Autodesk Inventor part; units mm, degrees
(part 2 of 2)
  line L223 (5.6866, -31.9003) -> (4.2323, -29.1462)
  line L224 (4.2323, -29.1462) -> (3.6335, -32.1998)
  line L225 (3.6335, -32.1998) -> (2.9735, -32.296)
  line L226 (-1.0989, -28.5985) -> (2.0334, -28.5439)
  line L227 (2.0334, -28.5439) -> (2.046, -29.2642)
  spline S287 degree 2 poles (2.046, -29.2642) (1.714, -29.587) (1.1233, -30.1861) (0.8407, -30.5081) knots 0 0 0 1 2 2 2
  spline S288 degree 2 poles (0.8407, -30.5081) (0.2715, -31.1562) (-0.1391, -31.9291) (-0.132, -32.3366) knots 0 0 0 1 2 2 2
  spline S289 degree 2 poles (-0.132, -32.3366) (-0.1283, -32.5507) (0.009, -32.8694) (0.1302, -32.9703) knots 0 0 0 1 2 2 2
  spline S290 degree 2 poles (0.1302, -32.9703) (0.2514, -33.0711) (0.566, -33.1685) (0.7553, -33.1652) knots 0 0 0 1 2 2 2
  spline S291 degree 2 poles (0.7553, -33.1652) (0.9364, -33.1621) (1.3053, -33.065) (1.4728, -32.9921) knots 0 0 0 1 2 2 2
  spline S292 degree 2 poles (1.4728, -32.9921) (1.6159, -32.932) (1.8806, -32.7627) (1.9619, -32.7036) knots 0 0 0 1 2 2 2
  line L228 (1.9619, -32.7036) -> (1.9989, -32.703)
  line L229 (1.9989, -32.703) -> (2.0115, -33.4274)
  spline S293 degree 2 poles (2.0115, -33.4274) (1.8034, -33.534) (1.0537, -33.7488) (0.7162, -33.7547) knots 0 0 0 1 2 2 2
  spline S294 degree 2 poles (0.7162, -33.7547) (0.0041, -33.7671) (-0.8117, -33.0278) (-0.8229, -32.3857) knots 0 0 0 1 2 2 2
  spline S295 degree 2 poles (-0.8229, -32.3857) (-0.8281, -32.0853) (-0.6969, -31.5807) (-0.5772, -31.3645) knots 0 0 0 1 2 2 2
  spline S296 degree 2 poles (-0.5772, -31.3645) (-0.4576, -31.1401) (-0.1071, -30.6975) (0.0868, -30.4841) knots 0 0 0 1 2 2 2
  spline S297 degree 2 poles (0.0868, -30.4841) (0.4018, -30.1287) (1.1749, -29.3659) (1.4057, -29.1436) knots 0 0 0 1 2 2 2
  line L230 (1.4057, -29.1436) -> (-1.0886, -29.1871)
  line L231 (-1.0886, -29.1871) -> (-1.0989, -28.5985)
  spline S298 degree 2 poles (-5.2095, -30.7189) (-5.0516, -29.3613) (-4.1145, -28.1813) (-3.2926, -28.2769) knots 0 0 0 1 2 2 2
  spline S299 degree 2 poles (-3.2926, -28.2769) (-2.4584, -28.3739) (-1.8281, -29.761) (-1.9827, -31.09) knots 0 0 0 1 2 2 2
  spline S300 degree 2 poles (-1.9827, -31.09) (-2.1415, -32.4558) (-3.0776, -33.6275) (-3.9037, -33.5315) knots 0 0 0 1 2 2 2
  spline S301 degree 2 poles (-3.9037, -33.5315) (-4.7337, -33.4349) (-5.3626, -32.0356) (-5.2095, -30.7189) knots 0 0 0 1 2 2 2
  spline S302 degree 2 poles (-4.1638, -29.2822) (-4.2909, -29.5202) (-4.4621, -30.2794) (-4.5225, -30.7988) knots 0 0 0 1 2 2 2
  spline S303 degree 2 poles (-4.5225, -30.7988) (-4.5829, -31.3181) (-4.59, -32.0923) (-4.5178, -32.3618) knots 0 0 0 1 2 2 2
  spline S304 degree 2 poles (-4.5178, -32.3618) (-4.4455, -32.6313) (-4.1207, -32.9384) (-3.8385, -32.9712) knots 0 0 0 1 2 2 2
  spline S305 degree 2 poles (-3.8385, -32.9712) (-3.5564, -33.0041) (-3.1615, -32.7806) (-3.0243, -32.5272) knots 0 0 0 1 2 2 2
  spline S306 degree 2 poles (-3.0243, -32.5272) (-2.8921, -32.2814) (-2.7272, -31.5049) (-2.6696, -31.0101) knots 0 0 0 1 2 2 2
  spline S307 degree 2 poles (-2.6696, -31.0101) (-2.6078, -30.4785) (-2.5905, -29.7594) (-2.6645, -29.469) knots 0 0 0 1 2 2 2
  spline S308 degree 2 poles (-2.6645, -29.469) (-2.7322, -29.1958) (-3.0633, -28.8714) (-3.3577, -28.8371) knots 0 0 0 1 2 2 2
  spline S309 degree 2 poles (-3.3577, -28.8371) (-3.6358, -28.8048) (-4.0306, -29.0283) (-4.1638, -29.2822) knots 0 0 0 1 2 2 2
  line L232 (-8.5894, -27.3003) -> (-5.5532, -28.0722)
  line L233 (-5.5532, -28.0722) -> (-5.7307, -28.7704)
  spline S310 degree 2 poles (-5.7307, -28.7704) (-6.136, -28.9945) (-6.8636, -29.4169) (-7.221, -29.6531) knots 0 0 0 1 2 2 2
  spline S311 degree 2 poles (-7.221, -29.6531) (-7.9407, -30.1285) (-8.5404, -30.7661) (-8.6408, -31.1611) knots 0 0 0 1 2 2 2
  spline S312 degree 2 poles (-8.6408, -31.1611) (-8.6936, -31.3685) (-8.645, -31.7122) (-8.5547, -31.8414) knots 0 0 0 1 2 2 2
  spline S313 degree 2 poles (-8.5547, -31.8414) (-8.4643, -31.9705) (-8.1865, -32.1474) (-8.0029, -32.194) knots 0 0 0 1 2 2 2
  spline S314 degree 2 poles (-8.0029, -32.194) (-7.8274, -32.2387) (-7.446, -32.2422) (-7.2652, -32.216) knots 0 0 0 1 2 2 2
  spline S315 degree 2 poles (-7.2652, -32.216) (-7.1113, -32.1956) (-6.8114, -32.1019) (-6.7174, -32.0664) knots 0 0 0 1 2 2 2
  line L234 (-6.7174, -32.0664) -> (-6.6815, -32.0755)
  line L235 (-6.6815, -32.0755) -> (-6.86, -32.7777)
  spline S316 degree 2 poles (-6.86, -32.7777) (-7.0889, -32.8257) (-7.8687, -32.8356) (-8.1959, -32.7524) knots 0 0 0 1 2 2 2
  spline S317 degree 2 poles (-8.1959, -32.7524) (-8.8861, -32.5769) (-9.4785, -31.649) (-9.3202, -31.0266) knots 0 0 0 1 2 2 2
  spline S318 degree 2 poles (-9.3202, -31.0266) (-9.2462, -30.7353) (-8.9867, -30.283) (-8.8143, -30.106) knots 0 0 0 1 2 2 2
  spline S319 degree 2 poles (-8.8143, -30.106) (-8.6398, -29.921) (-8.1852, -29.5863) (-7.942, -29.4316) knots 0 0 0 1 2 2 2
  spline S320 degree 2 poles (-7.942, -29.4316) (-7.5445, -29.1715) (-6.5979, -28.6392) (-6.3167, -28.4855) knots 0 0 0 1 2 2 2
  line L236 (-6.3167, -28.4855) -> (-8.7345, -27.8708)
  line L237 (-8.7345, -27.8708) -> (-8.5894, -27.3003)
  spline S321 degree 2 poles (-13.1132, -28.2636) (-12.6035, -26.9955) (-11.3888, -26.1039) (-10.621, -26.4125) knots 0 0 0 1 2 2 2
  spline S322 degree 2 poles (-10.621, -26.4125) (-9.8418, -26.7257) (-9.599, -28.2298) (-10.098, -29.4712) knots 0 0 0 1 2 2 2
  spline S323 degree 2 poles (-10.098, -29.4712) (-10.6108, -30.7469) (-11.8224, -31.6309) (-12.5939, -31.3208) knots 0 0 0 1 2 2 2
  spline S324 degree 2 poles (-12.5939, -31.3208) (-13.3693, -31.0091) (-13.6076, -29.4935) (-13.1132, -28.2636) knots 0 0 0 1 2 2 2
  spline S325 degree 2 poles (-11.7262, -27.1529) (-11.9115, -27.349) (-12.2765, -28.0364) (-12.4715, -28.5215) knots 0 0 0 1 2 2 2
  spline S326 degree 2 poles (-12.4715, -28.5215) (-12.6665, -29.0066) (-12.8772, -29.7516) (-12.8784, -30.0306) knots 0 0 0 1 2 2 2
  spline S327 degree 2 poles (-12.8784, -30.0306) (-12.8797, -30.3097) (-12.6472, -30.6915) (-12.3836, -30.7975) knots 0 0 0 1 2 2 2
  spline S328 degree 2 poles (-12.3836, -30.7975) (-12.1201, -30.9034) (-11.6803, -30.7918) (-11.4812, -30.5834) knots 0 0 0 1 2 2 2
  spline S329 degree 2 poles (-11.4812, -30.5834) (-11.289, -30.3811) (-10.9254, -29.6754) (-10.7397, -29.2132) knots 0 0 0 1 2 2 2
  spline S330 degree 2 poles (-10.7397, -29.2132) (-10.5401, -28.7167) (-10.334, -28.0275) (-10.3289, -27.7278) knots 0 0 0 1 2 2 2
  spline S331 degree 2 poles (-10.3289, -27.7278) (-10.3224, -27.4465) (-10.5564, -27.0463) (-10.8314, -26.9358) knots 0 0 0 1 2 2 2
  spline S332 degree 2 poles (-10.8314, -26.9358) (-11.0911, -26.8314) (-11.5309, -26.943) (-11.7262, -27.1529) knots 0 0 0 1 2 2 2
  line L238 (-24.6036, 2.7427) -> (-24.6056, 2.7098)
  spline S333 degree 2 poles (-24.6056, 2.7098) (-24.6436, 2.6255) (-24.7201, 2.3083) (-24.7276, 2.1809) knots 0 0 0 1 2 2 2
  spline S334 degree 2 poles (-24.7276, 2.1809) (-24.7514, 1.7782) (-24.4102, 1.4116) (-23.9335, 1.3834) knots 0 0 0 1 2 2 2
  line L239 (-23.9335, 1.3834) -> (-23.8061, 1.3759)
  line L240 (-23.8061, 1.3759) -> (-23.7434, 2.4361)
  line L241 (-23.7434, 2.4361) -> (-23.2133, 2.4047)
  line L242 (-23.2133, 2.4047) -> (-23.2748, 1.365)
  line L243 (-23.2748, 1.365) -> (-19.9995, 1.1712)
  line L244 (-19.9995, 1.1712) -> (-20.0375, 0.5301)
  line L245 (-20.0375, 0.5301) -> (-23.3127, 0.724)
  line L246 (-23.3127, 0.724) -> (-23.3383, 0.2925)
  line L247 (-23.3383, 0.2925) -> (-23.8684, 0.3238)
  line L248 (-23.8684, 0.3238) -> (-23.8429, 0.7553)
  line L249 (-23.8429, 0.7553) -> (-23.9703, 0.7629)
  spline S335 degree 2 poles (-23.9703, 0.7629) (-24.6524, 0.8032) (-25.3283, 1.5072) (-25.2918, 2.1236) knots 0 0 0 1 2 2 2
  spline S336 degree 2 poles (-25.2918, 2.1236) (-25.2814, 2.3003) (-25.2242, 2.6392) (-25.1913, 2.7775) knots 0 0 0 1 2 2 2
  line L250 (-25.1913, 2.7775) -> (-24.6036, 2.7427)
  line L251 (-19.7335, 3.4706) -> (-19.8346, 2.8364)
  line L252 (-19.8346, 2.8364) -> (-23.5991, 3.4365)
  line L253 (-23.5991, 3.4365) -> (-23.498, 4.0707)
  line L254 (-23.498, 4.0707) -> (-19.7335, 3.4706)
  line L255 (-24.117, 4.2152) -> (-24.2317, 3.4956)
  line L256 (-24.2317, 3.4956) -> (-24.8902, 3.6006)
  line L257 (-24.8902, 3.6006) -> (-24.7755, 4.3201)
  line L258 (-24.7755, 4.3201) -> (-24.117, 4.2152)
  line L259 (-19.3946, 5.0304) -> (-19.5458, 4.4063)
  line L260 (-19.5458, 4.4063) -> (-24.703, 5.6561)
  line L261 (-24.703, 5.6561) -> (-24.5517, 6.2802)
  line L262 (-24.5517, 6.2802) -> (-19.3946, 5.0304)
  spline S337 degree 2 poles (-18.5023, 7.4594) (-18.832, 6.607) (-20.1504, 6.04) (-21.0334, 6.3816) knots 0 0 0 1 2 2 2
  spline S338 degree 2 poles (-21.0334, 6.3816) (-21.9012, 6.7172) (-22.5781, 8.0252) (-22.2945, 8.7585) knots 0 0 0 1 2 2 2
  spline S339 degree 2 poles (-22.2945, 8.7585) (-22.1668, 9.0887) (-21.7773, 9.5251) (-21.501, 9.6345) knots 0 0 0 1 2 2 2
  spline S340 degree 2 poles (-21.501, 9.6345) (-21.2232, 9.7478) (-20.5571, 9.7241) (-20.1309, 9.5592) knots 0 0 0 1 2 2 2
  line L263 (-20.1309, 9.5592) -> (-19.8046, 9.433)
  line L264 (-19.8046, 9.433) -> (-20.7566, 6.9719)
  spline S341 degree 2 poles (-20.7566, 6.9719) (-20.1384, 6.7328) (-19.2413, 7.1008) (-19.0274, 7.6537) knots 0 0 0 1 2 2 2
  spline S342 degree 2 poles (-19.0274, 7.6537) (-18.9516, 7.8495) (-18.8929, 8.2637) (-18.9026, 8.4441) knots 0 0 0 1 2 2 2
  spline S343 degree 2 poles (-18.9026, 8.4441) (-18.917, 8.635) (-18.9653, 8.9097) (-18.9985, 9.0064) knots 0 0 0 1 2 2 2
  line L265 (-18.9985, 9.0064) -> (-18.9851, 9.0409)
  line L266 (-18.9851, 9.0409) -> (-18.3324, 8.7885)
  spline S344 degree 2 poles (-18.3324, 8.7885) (-18.3303, 8.6685) (-18.3292, 8.3061) (-18.3422, 8.1699) knots 0 0 0 1 2 2 2
  spline S345 degree 2 poles (-18.3422, 8.1699) (-18.3591, 7.9778) (-18.4191, 7.6744) (-18.5023, 7.4594) knots 0 0 0 1 2 2 2
  spline S346 degree 2 poles (-20.4872, 9.0261) (-20.7321, 9.112) (-21.1239, 9.1488) (-21.2801, 9.0988) knots 0 0 0 1 2 2 2
  spline S347 degree 2 poles (-21.2801, 9.0988) (-21.4545, 9.0472) (-21.7228, 8.7758) (-21.8164, 8.5339) knots 0 0 0 1 2 2 2
  spline S348 degree 2 poles (-21.8164, 8.5339) (-21.9085, 8.2958) (-21.8956, 7.9068) (-21.8109, 7.7152) knots 0 0 0 1 2 2 2
  spline S349 degree 2 poles (-21.8109, 7.7152) (-21.7208, 7.5258) (-21.4325, 7.2554) (-21.2134, 7.1486) knots 0 0 0 1 2 2 2
  line L267 (-21.2134, 7.1486) -> (-20.4872, 9.0261)
  line L268 (-17.161, 10.345) -> (-17.5675, 9.6386)
  line L269 (-17.5675, 9.6386) -> (-18.4096, 10.1231)
  line L270 (-18.4096, 10.1231) -> (-18.003, 10.8296)
  line L271 (-18.003, 10.8296) -> (-17.161, 10.345)
  line L272 (-19.623, 11.7618) -> (-20.0295, 11.0553)
  line L273 (-20.0295, 11.0553) -> (-20.8716, 11.5398)
  line L274 (-20.8716, 11.5398) -> (-20.465, 12.2463)
  line L275 (-20.465, 12.2463) -> (-19.623, 11.7618)
  spline S350 degree 2 poles (-14.6344, 12.8419) (-14.5674, 12.8679) (-14.3254, 12.9806) (-14.1854, 13.0675) knots 0 0 0 1 2 2 2
  spline S351 degree 2 poles (-14.1854, 13.0675) (-14.0279, 13.1602) (-13.777, 13.334) (-13.6514, 13.4588) knots 0 0 0 1 2 2 2
  spline S352 degree 2 poles (-13.6514, 13.4588) (-13.4412, 13.6677) (-13.2594, 14.0688) (-13.2763, 14.2494) knots 0 0 0 1 2 2 2
  spline S353 degree 2 poles (-13.2763, 14.2494) (-13.2961, 14.427) (-13.493, 14.7478) (-13.6584, 14.9143) knots 0 0 0 1 2 2 2
  line L276 (-13.6584, 14.9143) -> (-13.8934, 15.1508)
  spline S354 degree 2 poles (-13.8934, 15.1508) (-13.9178, 14.8074) (-14.1203, 14.3045) (-14.386, 14.0404) knots 0 0 0 1 2 2 2
  spline S355 degree 2 poles (-14.386, 14.0404) (-14.8474, 13.582) (-16.0754, 13.7256) (-16.7167, 14.371) knots 0 0 0 1 2 2 2
  spline S356 degree 2 poles (-16.7167, 14.371) (-17.0503, 14.7068) (-17.377, 15.4152) (-17.4021, 15.7559) knots 0 0 0 1 2 2 2
  spline S357 degree 2 poles (-17.4021, 15.7559) (-17.4215, 16.0791) (-17.1925, 16.6838) (-16.9705, 16.9043) knots 0 0 0 1 2 2 2
  spline S358 degree 2 poles (-16.9705, 16.9043) (-16.7603, 17.1132) (-16.355, 17.3186) (-16.1103, 17.3819) knots 0 0 0 1 2 2 2
  line L277 (-16.1103, 17.3819) -> (-16.1971, 17.5219)
  line L278 (-16.1971, 17.5219) -> (-15.7679, 17.9484)
  line L279 (-15.7679, 17.9484) -> (-13.3886, 15.5538)
  spline S359 degree 2 poles (-13.3886, 15.5538) (-12.7038, 14.8646) (-12.6641, 13.6274) (-13.2802, 13.0151) knots 0 0 0 1 2 2 2
  spline S360 degree 2 poles (-13.2802, 13.0151) (-13.4788, 12.8178) (-13.9573, 12.47) (-14.1877, 12.3456) knots 0 0 0 1 2 2 2
  line L280 (-14.1877, 12.3456) -> (-14.6578, 12.8187)
  line L281 (-14.6578, 12.8187) -> (-14.6344, 12.8419)
  line L282 (-14.2648, 15.5246) -> (-15.7418, 17.011)
  spline S361 degree 2 poles (-15.7418, 17.011) (-15.9924, 16.9245) (-16.3482, 16.7102) (-16.4913, 16.568) knots 0 0 0 1 2 2 2
  spline S362 degree 2 poles (-16.4913, 16.568) (-16.8359, 16.2256) (-16.7282, 15.3229) (-16.2552, 14.8469) knots 0 0 0 1 2 2 2
  spline S363 degree 2 poles (-16.2552, 14.8469) (-15.8084, 14.3972) (-15.0404, 14.2259) (-14.7017, 14.5625) knots 0 0 0 1 2 2 2
  spline S364 degree 2 poles (-14.7017, 14.5625) (-14.5235, 14.7395) (-14.289, 15.2511) (-14.2648, 15.5246) knots 0 0 0 1 2 2 2
  spline S365 degree 2 poles (-10.9409, 16.6815) (-11.6979, 16.1695) (-13.1042, 16.4559) (-13.6346, 17.2403) knots 0 0 0 1 2 2 2
  spline S366 degree 2 poles (-13.6346, 17.2403) (-14.1558, 18.011) (-13.9657, 19.4714) (-13.3144, 19.9119) knots 0 0 0 1 2 2 2
  spline S367 degree 2 poles (-13.3144, 19.9119) (-13.0211, 20.1102) (-12.4522, 20.2464) (-12.1629, 20.1787) knots 0 0 0 1 2 2 2
  spline S368 degree 2 poles (-12.1629, 20.1787) (-11.8702, 20.1133) (-11.3366, 19.7138) (-11.0806, 19.3352) knots 0 0 0 1 2 2 2
  line L283 (-11.0806, 19.3352) -> (-10.8846, 19.0454)
  line L284 (-10.8846, 19.0454) -> (-13.0705, 17.5671)
  spline S369 degree 2 poles (-13.0705, 17.5671) (-12.6992, 17.0181) (-11.7524, 16.8086) (-11.2613, 17.1407) knots 0 0 0 1 2 2 2
  spline S370 degree 2 poles (-11.2613, 17.1407) (-11.0874, 17.2583) (-10.8029, 17.565) (-10.708, 17.7187) knots 0 0 0 1 2 2 2
  spline S371 degree 2 poles (-10.708, 17.7187) (-10.6109, 17.8837) (-10.4938, 18.1368) (-10.4659, 18.2352) knots 0 0 0 1 2 2 2
  line L285 (-10.4659, 18.2352) -> (-10.4352, 18.256)
  line L286 (-10.4352, 18.256) -> (-10.0432, 17.6762)
  spline S372 degree 2 poles (-10.0432, 17.6762) (-10.1099, 17.5765) (-10.3157, 17.2782) (-10.4041, 17.1738) knots 0 0 0 1 2 2 2
  spline S373 degree 2 poles (-10.4041, 17.1738) (-10.5275, 17.0256) (-10.7499, 16.8107) (-10.9409, 16.6815) knots 0 0 0 1 2 2 2
  spline S374 degree 2 poles (-11.6774, 19.1007) (-11.8295, 19.3109) (-12.1303, 19.5646) (-12.287, 19.6127) knots 0 0 0 1 2 2 2
  spline S375 degree 2 poles (-12.287, 19.6127) (-12.4598, 19.6698) (-12.835, 19.5999) (-13.0499, 19.4547) knots 0 0 0 1 2 2 2
  spline S376 degree 2 poles (-13.0499, 19.4547) (-13.2613, 19.3117) (-13.4726, 18.9849) (-13.5124, 18.7791) knots 0 0 0 1 2 2 2
  spline S377 degree 2 poles (-13.5124, 18.7791) (-13.5464, 18.5722) (-13.4639, 18.1857) (-13.3449, 17.9729) knots 0 0 0 1 2 2 2
  line L287 (-13.3449, 17.9729) -> (-11.6774, 19.1007)
  spline S378 degree 2 poles (-7.4887, 19.0308) (-7.5373, 18.9466) (-7.6964, 18.6525) (-7.7848, 18.5465) knots 0 0 0 1 2 2 2
  spline S379 degree 2 poles (-7.7848, 18.5465) (-7.9032, 18.396) (-8.1558, 18.1823) (-8.4199, 18.0669) knots 0 0 0 1 2 2 2
  spline S380 degree 2 poles (-8.4199, 18.0669) (-8.6349, 17.973) (-9.0943, 17.9655) (-9.3057, 18.0484) knots 0 0 0 1 2 2 2
  spline S381 degree 2 poles (-9.3057, 18.0484) (-9.5079, 18.1307) (-9.8623, 18.4791) (-9.9644, 18.713) knots 0 0 0 1 2 2 2
  spline S382 degree 2 poles (-9.9644, 18.713) (-10.1226, 19.0752) (-10.0412, 19.7217) (-9.7735, 20.0138) knots 0 0 0 1 2 2 2
  spline S383 degree 2 poles (-9.7735, 20.0138) (-9.5385, 20.2782) (-8.7833, 20.7294) (-8.3308, 20.9585) knots 0 0 0 1 2 2 2
  line L288 (-8.3308, 20.9585) -> (-8.3802, 21.0717)
  spline S384 degree 2 poles (-8.3802, 21.0717) (-8.4692, 21.2754) (-8.7041, 21.4738) (-8.8486, 21.496) knots 0 0 0 1 2 2 2
  spline S385 degree 2 poles (-8.8486, 21.496) (-8.9931, 21.5182) (-9.3373, 21.4218) (-9.5108, 21.346) knots 0 0 0 1 2 2 2
  spline S386 degree 2 poles (-9.5108, 21.346) (-9.7145, 21.257) (-10.2126, 20.8957) (-10.4369, 20.6584) knots 0 0 0 1 2 2 2
  line L289 (-10.4369, 20.6584) -> (-10.4708, 20.6436)
  line L290 (-10.4708, 20.6436) -> (-10.7329, 21.2434)
  spline S387 degree 2 poles (-10.7329, 21.2434) (-10.5904, 21.3596) (-10.0325, 21.738) (-9.7345, 21.8682) knots 0 0 0 1 2 2 2
  spline S388 degree 2 poles (-9.7345, 21.8682) (-9.3723, 22.0264) (-8.8287, 22.1291) (-8.5682, 22.0677) knots 0 0 0 1 2 2 2
  spline S389 degree 2 poles (-8.5682, 22.0677) (-8.3132, 22.0084) (-7.9252, 21.6343) (-7.7818, 21.3061) knots 0 0 0 1 2 2 2
  line L291 (-7.7818, 21.3061) -> (-6.7387, 18.9181)
  line L292 (-6.7387, 18.9181) -> (-7.3272, 18.6611)
  line L293 (-7.3272, 18.6611) -> (-7.4887, 19.0308)
  line L294 (-7.7029, 19.5212) -> (-8.1264, 20.4907)
  spline S390 degree 2 poles (-8.1264, 20.4907) (-8.3295, 20.3796) (-8.939, 20.0369) (-9.1126, 19.8892) knots 0 0 0 1 2 2 2
  spline S391 degree 2 poles (-9.1126, 19.8892) (-9.3152, 19.7154) (-9.4905, 19.2839) (-9.3752, 19.0198) knots 0 0 0 1 2 2 2
  spline S392 degree 2 poles (-9.3752, 19.0198) (-9.2434, 18.718) (-8.7704, 18.5607) (-8.4459, 18.7025) knots 0 0 0 1 2 2 2
  spline S393 degree 2 poles (-8.4459, 18.7025) (-8.1705, 18.8228) (-7.8217, 19.2582) (-7.7029, 19.5212) knots 0 0 0 1 2 2 2
  line L295 (-4.717, 22.706) -> (-4.7489, 22.6976)
  spline S394 degree 2 poles (-4.7489, 22.6976) (-4.8258, 22.6986) (-4.9831, 22.6657) (-5.0906, 22.6373) knots 0 0 0 1 2 2 2
  spline S395 degree 2 poles (-5.0906, 22.6373) (-5.3414, 22.5712) (-5.7773, 22.2222) (-5.9435, 21.9485) knots 0 0 0 1 2 2 2
  line L296 (-5.9435, 21.9485) -> (-5.2541, 19.3331)
  line L297 (-5.2541, 19.3331) -> (-5.8751, 19.1694)
  line L298 (-5.8751, 19.1694) -> (-6.8468, 22.8556)
  line L299 (-6.8468, 22.8556) -> (-6.2258, 23.0193)
  line L300 (-6.2258, 23.0193) -> (-6.081, 22.4699)
  spline S396 degree 2 poles (-6.081, 22.4699) (-5.8224, 22.8617) (-5.3819, 23.2417) (-5.1431, 23.3047) knots 0 0 0 1 2 2 2
  spline S397 degree 2 poles (-5.1431, 23.3047) (-5.0475, 23.3299) (-4.9499, 23.3471) (-4.887, 23.3509) knots 0 0 0 1 2 2 2
  line L301 (-4.887, 23.3509) -> (-4.717, 22.706)
  line L302 (-0.4579, 20.1023) -> (-3.384, 19.7837)
  line L303 (-3.384, 19.7837) -> (-3.9339, 24.8339)
  line L304 (-3.9339, 24.8339) -> (-3.2628, 24.9069)
  line L305 (-3.2628, 24.9069) -> (-2.7779, 20.4543)
  line L306 (-2.7779, 20.4543) -> (-0.523, 20.6998)
  line L307 (-0.523, 20.6998) -> (-0.4579, 20.1023)
  spline S398 degree 2 poles (3.2846, 21.7592) (3.2149, 20.7985) (2.2151, 19.8184) (1.4432, 19.8744) knots 0 0 0 1 2 2 2
  spline S399 degree 2 poles (1.4432, 19.8744) (0.6508, 19.9319) (-0.1783, 21.0775) (-0.111, 22.0055) knots 0 0 0 1 2 2 2
  spline S400 degree 2 poles (-0.111, 22.0055) (-0.0419, 22.958) (0.9707, 23.9454) (1.7344, 23.89) knots 0 0 0 1 2 2 2
  spline S401 degree 2 poles (1.7344, 23.89) (2.5063, 23.834) (3.3539, 22.7159) (3.2846, 21.7592) knots 0 0 0 1 2 2 2
  spline S402 degree 2 poles (2.6235, 21.8072) (2.6771, 22.5462) (2.1913, 23.3038) (1.6945, 23.3398) knots 0 0 0 1 2 2 2
  spline S403 degree 2 poles (1.6945, 23.3398) (1.1977, 23.3758) (0.6036, 22.6966) (0.55, 21.9575) knots 0 0 0 1 2 2 2
  spline S404 degree 2 poles (0.55, 21.9575) (0.4979, 21.239) (0.9863, 20.4606) (1.4831, 20.4246) knots 0 0 0 1 2 2 2
  spline S405 degree 2 poles (1.4831, 20.4246) (1.9758, 20.3889) (2.5705, 21.0763) (2.6235, 21.8072) knots 0 0 0 1 2 2 2
  spline S406 degree 2 poles (5.2345, 19.2518) (4.8513, 19.3484) (4.276, 19.744) (4.1088, 20.0409) knots 0 0 0 1 2 2 2
  spline S407 degree 2 poles (4.1088, 20.0409) (3.9407, 20.3337) (3.8724, 21.1237) (3.9952, 21.6107) knots 0 0 0 1 2 2 2
  spline S408 degree 2 poles (3.9952, 21.6107) (4.118, 22.0976) (4.5566, 22.7427) (4.8366, 22.9269) knots 0 0 0 1 2 2 2
  spline S409 degree 2 poles (4.8366, 22.9269) (5.1175, 23.115) (5.8336, 23.2104) (6.2088, 23.1158) knots 0 0 0 1 2 2 2
  spline S410 degree 2 poles (6.2088, 23.1158) (6.5122, 23.0393) (7.0357, 22.7247) (7.2271, 22.5576) knots 0 0 0 1 2 2 2
  line L308 (7.2271, 22.5576) -> (7.051, 21.8591)
  line L309 (7.051, 21.8591) -> (7.015, 21.8681)
  spline S411 degree 2 poles (7.015, 21.8681) (6.9613, 21.9411) (6.7899, 22.1371) (6.6614, 22.2502) knots 0 0 0 1 2 2 2
  spline S412 degree 2 poles (6.6614, 22.2502) (6.5457, 22.3473) (6.2196, 22.5357) (6.06, 22.576) knots 0 0 0 1 2 2 2
  spline S413 degree 2 poles (6.06, 22.576) (5.577, 22.6977) (4.806, 22.1152) (4.6379, 21.4486) knots 0 0 0 1 2 2 2
  spline S414 degree 2 poles (4.6379, 21.4486) (4.4738, 20.7979) (4.8564, 19.9245) (5.3594, 19.7977) knots 0 0 0 1 2 2 2
  spline S415 degree 2 poles (5.3594, 19.7977) (5.6628, 19.7212) (6.277, 19.8338) (6.5379, 19.976) knots 0 0 0 1 2 2 2
  line L310 (6.5379, 19.976) -> (6.5739, 19.967)
  line L311 (6.5739, 19.967) -> (6.3977, 19.2684)
  spline S416 degree 2 poles (6.3977, 19.2684) (6.2948, 19.2477) (5.9842, 19.1944) (5.8654, 19.1946) knots 0 0 0 1 2 2 2
  spline S417 degree 2 poles (5.8654, 19.1946) (5.6936, 19.187) (5.4301, 19.2025) (5.2345, 19.2518) knots 0 0 0 1 2 2 2
  line L312 (9.7814, 17.5848) -> (9.0087, 17.9242)
  line L313 (9.0087, 17.9242) -> (8.4522, 20.1785)
  line L314 (8.4522, 20.1785) -> (8.1192, 20.055)
  line L315 (8.1192, 20.055) -> (7.4784, 18.5964)
  line L316 (7.4784, 18.5964) -> (6.8905, 18.8546)
  line L317 (6.8905, 18.8546) -> (9.0245, 23.713)
  line L318 (9.0245, 23.713) -> (9.6125, 23.4547)
  line L319 (9.6125, 23.4547) -> (8.3642, 20.6128)
  line L320 (8.3642, 20.6128) -> (10.391, 21.4806)
  line L321 (10.391, 21.4806) -> (11.1222, 21.1594)
  line L322 (11.1222, 21.1594) -> (9.0492, 20.3299)
  line L323 (9.0492, 20.3299) -> (9.7814, 17.5848)
  line L324 (10.8701, 16.8332) -> (10.1766, 17.2615)
  line L325 (10.1766, 17.2615) -> (10.6871, 18.0881)
  line L326 (10.6871, 18.0881) -> (11.3806, 17.6598)
  line L327 (11.3806, 17.6598) -> (10.8701, 16.8332)
  line L328 (12.3144, 15.8054) -> (11.8015, 16.192)
  line L329 (11.8015, 16.192) -> (14.0959, 19.2362)
  line L330 (14.0959, 19.2362) -> (14.6088, 18.8497)
  line L331 (14.6088, 18.8497) -> (12.3144, 15.8054)
  line L332 (15.0265, 19.3287) -> (14.4446, 19.7673)
  line L333 (14.4446, 19.7673) -> (14.846, 20.2999)
  line L334 (14.846, 20.2999) -> (15.4279, 19.8613)
  line L335 (15.4279, 19.8613) -> (15.0265, 19.3287)
  spline S418 degree 2 poles (16.757, 14.4248) (16.0841, 13.747) (14.6438, 13.5875) (14.15, 14.0777) knots 0 0 0 1 2 2 2
  spline S419 degree 2 poles (14.15, 14.0777) (13.9484, 14.2778) (13.7316, 14.6787) (13.6666, 14.9347) knots 0 0 0 1 2 2 2
  line L336 (13.6666, 14.9347) -> (12.5413, 13.8011)
  line L337 (12.5413, 13.8011) -> (12.0855, 14.2536)
  line L338 (12.0855, 14.2536) -> (15.7603, 17.9551)
  line L339 (15.7603, 17.9551) -> (16.216, 17.5026)
  line L340 (16.216, 17.5026) -> (15.9347, 17.2192)
  spline S420 degree 2 poles (15.9347, 17.2192) (16.2579, 17.2059) (16.8757, 16.9985) (17.1182, 16.7578) knots 0 0 0 1 2 2 2
  spline S421 degree 2 poles (17.1182, 16.7578) (17.5827, 16.2966) (17.3719, 15.0441) (16.757, 14.4248) knots 0 0 0 1 2 2 2
  spline S422 degree 2 poles (16.2344, 14.8392) (16.6956, 15.3037) (16.9081, 16.1079) (16.578, 16.4356) knots 0 0 0 1 2 2 2
  spline S423 degree 2 poles (16.578, 16.4356) (16.3851, 16.627) (15.8518, 16.8143) (15.5577, 16.8395) knots 0 0 0 1 2 2 2
  line L341 (15.5577, 16.8395) -> (14.0321, 15.3028)
  spline S424 degree 2 poles (14.0321, 15.3028) (14.1262, 15.0411) (14.3165, 14.7245) (14.4801, 14.5621) knots 0 0 0 1 2 2 2
  spline S425 degree 2 poles (14.4801, 14.5621) (14.8336, 14.2111) (15.7414, 14.3425) (16.2344, 14.8392) knots 0 0 0 1 2 2 2
  spline S426 degree 2 poles (16.3391, 11.4727) (16.0291, 11.8937) (16.1608, 12.7217) (16.6813, 13.1049) knots 0 0 0 1 2 2 2
  line L342 (16.6813, 13.1049) -> (18.3819, 14.357)
  line L343 (18.3819, 14.357) -> (18.1256, 14.7051)
  line L344 (18.1256, 14.7051) -> (18.5533, 15.02)
  line L345 (18.5533, 15.02) -> (18.8095, 14.6719)
  line L346 (18.8095, 14.6719) -> (19.6914, 15.3211)
  line L347 (19.6914, 15.3211) -> (20.0721, 14.804)
  line L348 (20.0721, 14.804) -> (19.1903, 14.1547)
  line L349 (19.1903, 14.1547) -> (19.8908, 13.2033)
  line L350 (19.8908, 13.2033) -> (19.4632, 12.8884)
  line L351 (19.4632, 12.8884) -> (18.7627, 13.8399)
  line L352 (18.7627, 13.8399) -> (17.3007, 12.7635)
  spline S427 degree 2 poles (17.3007, 12.7635) (17.0687, 12.5926) (16.8256, 12.3881) (16.7577, 12.2512) knots 0 0 0 1 2 2 2
  spline S428 degree 2 poles (16.7577, 12.2512) (16.6957, 12.134) (16.7534, 11.8544) (16.8852, 11.6754) knots 0 0 0 1 2 2 2
  spline S429 degree 2 poles (16.8852, 11.6754) (16.9779, 11.5494) (17.2275, 11.3702) (17.2897, 11.3342) knots 0 0 0 1 2 2 2
  line L353 (17.2897, 11.3342) -> (17.3117, 11.3044)
  line L354 (17.3117, 11.3044) -> (16.8476, 10.9627)
  spline S430 degree 2 poles (16.8476, 10.9627) (16.7004, 11.0792) (16.4343, 11.3434) (16.3391, 11.4727) knots 0 0 0 1 2 2 2
  spline S431 degree 2 poles (-14.696, 4.2549) (-14.3711, 4.2011) (-13.8246, 3.8728) (-13.6558, 3.6321) knots 0 0 0 1 2 2 2
  spline S432 degree 2 poles (-13.6558, 3.6321) (-13.4429, 3.3298) (-13.2952, 2.5835) (-13.3839, 2.0474) knots 0 0 0 1 2 2 2
  line L355 (-13.3839, 2.0474) -> (-13.4773, 1.4829)
  line L356 (-13.4773, 1.4829) -> (-11.609, 1.1738)
  line L357 (-11.609, 1.1738) -> (-11.7192, 0.5077)
  line L358 (-11.7192, 0.5077) -> (-16.731, 1.3369)
  line L359 (-16.731, 1.3369) -> (-16.5227, 2.5959)
  spline S433 degree 2 poles (-16.5227, 2.5959) (-16.4488, 3.0427) (-16.1991, 3.644) (-15.993, 3.8561) knots 0 0 0 1 2 2 2
  spline S434 degree 2 poles (-15.993, 3.8561) (-15.7557, 4.1047) (-15.1144, 4.3241) (-14.696, 4.2549) knots 0 0 0 1 2 2 2
  spline S435 degree 2 poles (-14.7906, 3.557) (-15.0506, 3.6) (-15.4619, 3.4845) (-15.614, 3.3219) knots 0 0 0 1 2 2 2
  spline S436 degree 2 poles (-15.614, 3.3219) (-15.7458, 3.1809) (-15.901, 2.7726) (-15.9527, 2.4599) knots 0 0 0 1 2 2 2
  line L360 (-15.9527, 2.4599) -> (-16.0441, 1.9075)
  line L361 (-16.0441, 1.9075) -> (-14.0459, 1.5769)
  line L362 (-14.0459, 1.5769) -> (-13.9706, 2.0318)
  spline S437 degree 2 poles (-13.9706, 2.0318) (-13.9034, 2.438) (-13.9507, 2.959) (-14.0944, 3.1497) knots 0 0 0 1 2 2 2
  spline S438 degree 2 poles (-14.0944, 3.1497) (-14.2198, 3.3249) (-14.551, 3.5174) (-14.7906, 3.557) knots 0 0 0 1 2 2 2
  line L363 (-13.6035, 9.9505) -> (-10.0141, 5.9526)
  line L364 (-10.0141, 5.9526) -> (-10.3682, 5.3158)
  line L365 (-10.3682, 5.3158) -> (-15.6583, 6.2555)
  line L366 (-15.6583, 6.2555) -> (-15.3061, 6.8887)
  line L367 (-15.3061, 6.8887) -> (-10.9341, 6.0685)
  line L368 (-10.9341, 6.0685) -> (-13.9377, 9.3497)
  line L369 (-13.9377, 9.3497) -> (-13.6035, 9.9505)
  line L370 (-9.877, 10.6037) -> (-10.4575, 10.0316)
  line L371 (-10.4575, 10.0316) -> (-11.1395, 10.7236)
  line L372 (-11.1395, 10.7236) -> (-10.5589, 11.2957)
  line L373 (-10.5589, 11.2957) -> (-9.877, 10.6037)
  line L374 (-7.8832, 8.5805) -> (-8.4638, 8.0083)
  line L375 (-8.4638, 8.0083) -> (-9.1457, 8.7003)
  line L376 (-9.1457, 8.7003) -> (-8.5651, 9.2725)
  line L377 (-8.5651, 9.2725) -> (-7.8832, 8.5805)
  spline S439 degree 2 poles (-2.9651, 13.9665) (-2.5309, 12.6706) (-2.8774, 11.2042) (-3.662, 10.9413) knots 0 0 0 1 2 2 2
  spline S440 degree 2 poles (-3.662, 10.9413) (-4.4583, 10.6744) (-5.6185, 11.662) (-6.0436, 12.9306) knots 0 0 0 1 2 2 2
  spline S441 degree 2 poles (-6.0436, 12.9306) (-6.4805, 14.2343) (-6.1313, 15.6929) (-5.3428, 15.9571) knots 0 0 0 1 2 2 2
  spline S442 degree 2 poles (-5.3428, 15.9571) (-4.5504, 16.2226) (-3.3863, 15.2234) (-2.9651, 13.9665) knots 0 0 0 1 2 2 2
  spline S443 degree 2 poles (-3.3008, 12.2215) (-3.287, 12.491) (-3.4548, 13.251) (-3.6209, 13.7467) knots 0 0 0 1 2 2 2
  spline S444 degree 2 poles (-3.6209, 13.7467) (-3.787, 14.2425) (-4.1097, 14.9462) (-4.2897, 15.1595) knots 0 0 0 1 2 2 2
  spline S445 degree 2 poles (-4.2897, 15.1595) (-4.4697, 15.3727) (-4.8943, 15.5126) (-5.1636, 15.4223) knots 0 0 0 1 2 2 2
  spline S446 degree 2 poles (-5.1636, 15.4223) (-5.4329, 15.3321) (-5.6953, 14.962) (-5.7118, 14.6742) knots 0 0 0 1 2 2 2
  spline S447 degree 2 poles (-5.7118, 14.6742) (-5.727, 14.3956) (-5.5461, 13.6226) (-5.3878, 13.1503) knots 0 0 0 1 2 2 2
  spline S448 degree 2 poles (-5.3878, 13.1503) (-5.2178, 12.6429) (-4.9277, 11.9846) (-4.7373, 11.7532) knots 0 0 0 1 2 2 2
  spline S449 degree 2 poles (-4.7373, 11.7532) (-4.5599, 11.5348) (-4.1223, 11.3819) (-3.8412, 11.476) knots 0 0 0 1 2 2 2
  spline S450 degree 2 poles (-3.8412, 11.476) (-3.5758, 11.565) (-3.3134, 11.9351) (-3.3008, 12.2215) knots 0 0 0 1 2 2 2
  line L378 (1.6106, 11.643) -> (-1.5222, 11.6466)
  line L379 (-1.5222, 11.6466) -> (-1.5213, 12.367)
  spline S451 degree 2 poles (-1.5213, 12.367) (-1.1834, 12.6836) (-0.5817, 13.2716) (-0.2932, 13.5883) knots 0 0 0 1 2 2 2
  spline S452 degree 2 poles (-0.2932, 13.5883) (0.288, 14.2257) (0.7129, 14.9909) (0.7134, 15.3985) knots 0 0 0 1 2 2 2
  spline S453 degree 2 poles (0.7134, 15.3985) (0.7136, 15.6126) (0.5823, 15.9338) (0.463, 16.0369) knots 0 0 0 1 2 2 2
  spline S454 degree 2 poles (0.463, 16.0369) (0.3437, 16.1399) (0.031, 16.2432) (-0.1584, 16.2434) knots 0 0 0 1 2 2 2
  spline S455 degree 2 poles (-0.1584, 16.2434) (-0.3395, 16.2436) (-0.7101, 16.1535) (-0.879, 16.0837) knots 0 0 0 1 2 2 2
  spline S456 degree 2 poles (-0.879, 16.0837) (-1.0231, 16.0262) (-1.2909, 15.8619) (-1.3733, 15.8043) knots 0 0 0 1 2 2 2
  line L380 (-1.3733, 15.8043) -> (-1.4104, 15.8044)
  line L381 (-1.4104, 15.8044) -> (-1.4095, 16.5289)
  spline S457 degree 2 poles (-1.4095, 16.5289) (-1.1995, 16.6316) (-0.4459, 16.8324) (-0.1083, 16.832) knots 0 0 0 1 2 2 2
  spline S458 degree 2 poles (-0.1083, 16.832) (0.6039, 16.8312) (1.4058, 16.0769) (1.405, 15.4347) knots 0 0 0 1 2 2 2
  spline S459 degree 2 poles (1.405, 15.4347) (1.4047, 15.1342) (1.2641, 14.6322) (1.1404, 14.4182) knots 0 0 0 1 2 2 2
  spline S460 degree 2 poles (1.1404, 14.4182) (1.0166, 14.1961) (0.658, 13.7601) (0.4601, 13.5504) knots 0 0 0 1 2 2 2
  spline S461 degree 2 poles (0.4601, 13.5504) (0.1386, 13.2008) (-0.6485, 12.4525) (-0.8834, 12.2346) knots 0 0 0 1 2 2 2
  line L382 (-0.8834, 12.2346) -> (1.6113, 12.2317)
  line L383 (1.6113, 12.2317) -> (1.6106, 11.643)
  dimension "d181" = 57.15
  constraints: 1 centre point, 1 coincident, 1 other
  measures "d181" diameter of A0
extrude "Extrusion26" cut sketch "Sketch28" against normal blind 1.27
split "Split1" plane through (0, 0, 0) removes the side toward (0, 0, 1)
equation "\"d0\" = externalDiameter - 2 * printSpacing"
equation "\"d55\" = hexSize + 2 * printSpacing"
equation "\"d123\" = depthOfExternalSpline"
equation "\"d124\" = 0.5 * absPrintSpacingAngleDiff"
equation "\"d125\" = angleForSplineTooth"
equation "\"d126\" = thickness"
equation "\"internalDiameter\" = 50.8"
equation "\"externalDiameter\" = 76.2"
equation "\"pi\" = 3.141593"
equation "\"depthOfInternalSpline\" = 0.5 * widthOfInternalSpline"
equation "\"depthOfExternalSpline\" = 0.5 * widthOfExternalSpline"
equation "\"thickness\" = 9.525"
equation "\"hexSize\" = 12.7"
equation "\"printSpacing\" = 0.1905"
equation "\"holeDiameterForBushing\" = 50.8"
equation "\"printSpacingAngleDiff\" = -2deg"
equation "\"gapSpacing\" = 7.9375"
equation "\"oneHalfGapSpacing\" = 0.5 * gapSpacing"
equation "\"gapDepth\" = 7.14375"
equation "\"gapCircleDiameter\" = 63.5"
equation "\"shouldBoltSpaceing\" = 4.7625"
equation "\"oneHalfShouldBoltSpacing\" = 0.5 * shouldBoltSpaceing"
equation "\"absPrintSpacingAngleDiff\" = 2deg"
equation "\"angleForSplineTooth\" = 13deg"
equation "\"widthOfInternalSpline\" = 6.649704"
equation "\"widthOfExternalSpline\" = 9.974557"
body "Solid1"
